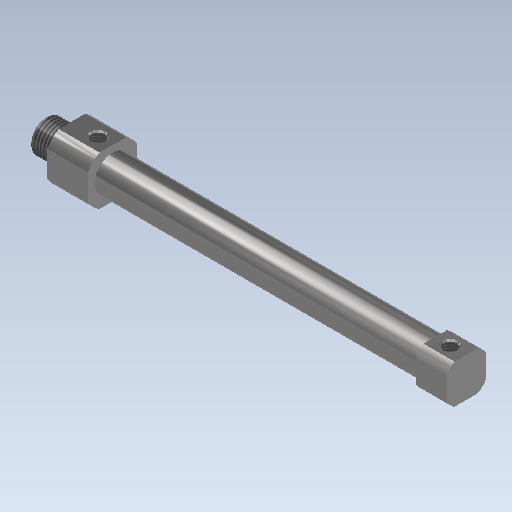
# Autodesk Inventor part: CJ2KB10-75Z(0)_BODY
Saved by Autodesk Inventor 2021.3 (Build 253353010, 353A)
## iProperties
Created: 2019-10-24
Part Number: CJ2KB10-75Z(0)_BODY
Material: ステンレス鋼
Catalog Web Link: www.cadenas.de
Description: CJ2K-Z_BODY-Air Cylinder/Non-rotating Rod Type: Double Acting, Single Rod
Vendor: SMC
Document SubType Name: Modeling
Designer: psadmin
Manufacturer: SMC
Mass: 57.0241 g
Surface Area: 82.6037 cm^2
Volume: 7.12801 cm^3
Density: 8 g/cm^3
Appearance: 半つや出し
Category: PARTsolutions
Company: SMC
PSOL_IDENT_0: {$CADENAS_DATA\23d-libs\smc_jp\actuator\standard_air_cylinder\cj2\cj2k_z\parts\cj2k_z_body.prj},256
PSOL_IDENT_1: {VTYP=3D},{NB=CJ2KB10-75Z(0)_BODY},{LINA=CJ2KB10-75Z_BODY},{NN=CJ2K-Z_BODY},{DATE=07.02.2019 07:32:0
PSOL_IDENT_2: 0},{GEOMDATE=05.03.2018 07:17:00},{VERSION=},{LINEID=370},{WBVAR=MAGNET,AUTOSWITCH,NUMBER,STROKE,POR
PSOL_IDENT_3: T,MOUNTING,OMSCXC3,OMSCXC51,THREAD},{WBNUMERIC=STROKE}  {NB=CJ2KB10-75Z(0)_BODY},{LINA=CJ2KB10-75Z_B
PSOL_IDENT_4: ODY},{KT=DUMMY},{ORDER=CJ2KB10-75Z},{BORE=10},{MOUNT=(B) Basic},{MAGNET=},{MOUNTX=B},{AUTOSWITCH=},{
PSOL_IDENT_5: NUMBER=},{STROKE=75},{SMAX=400},{PORT=},{PORTX='', '(-) Perpendicular', 'R', '(R) In-line'},{MOUNTIN
PSOL_IDENT_6: G=},{MOUNTINGX='','N/A'},{OMSCXC3=},{OMSCXC51=},{THREAD=0},{BA=15.0},{BB=12.0},{CA=17.0},{CB=14.0},{
PSOL_IDENT_7: CD=0.0},{CX=0.0},{F=8},{GA=8.0},{GB=5.0},{H=28},{KA=4.2},{NA=12.5},{NB1=9.5},{NDH8=10 0/-0.022},{NN=
PSOL_IDENT_8: M10x1.0},{NN1=10},{NN2=1.0},{R=0},{S=46},{U=0},{RAIL=off},{AUTOSWX='','N/A'},{SW=4.5},{SWX=4.5},{SW1=
PSOL_IDENT_9: 6.000},{SW2=2.000},{SW3=2.500},{SW4=1.500},{SW5=4.500},{SW6=0.500},{SW7=3.000},{SW8=3.500},{SW9=0.50
PSOL_IDENT_10: 0},{SWSIGNX= '','N/A' },{XC3= '','(-) None','-XC3AB','(XC3AB) Special Port Location (Rod port locati
PSOL_IDENT_11: on: A,Head port location: B)','-XC3AC','(XC3AC) Special Port Location (Rod port location: A,Head por
PSOL_IDENT_12: t location: C)','-XC3AD','(XC3AD) Special Port Location (Rod port location: A,Head port location: D)'
PSOL_IDENT_13: ,'-XC3BA','(XC3BA) Special Port Location (Rod port location: B,Head port location: A)','-XC3BB','(XC
PSOL_IDENT_14: 3BB) Special Port Location (Rod port location: B,Head port location: B)','-XC3BC','(XC3BC) Special P
PSOL_IDENT_15: ort Location (Rod port location: B,Head port location: C)','-XC3BD','(XC3BD) Special Port Location (
PSOL_IDENT_16: Rod port location: B,Head port location: D)','-XC3CA','(XC3CA) Special Port Location (Rod port locat
PSOL_IDENT_17: ion: C,Head port location: A)','-XC3CB','(XC3CB) Special Port Location (Rod port location: C,Head po
PSOL_IDENT_18: rt location: B)','-XC3CC','(XC3CC) Special Port Location (Rod port location: C,Head port location: C
PSOL_IDENT_19: )','-XC3CD','(XC3CD) Special Port Location (Rod port location: C,Head port location: D)','-XC3DA','(
PSOL_IDENT_20: XC3DA) Special Port Location (Rod port location: D,Head port location: A)','-XC3DB','(XC3DB) Special
PSOL_IDENT_21: Port Location (Rod port location: D,Head port location: B)','-XC3DC','(XC3DC) Special Port Location
PSOL_IDENT_22: (Rod port location: D,Head port location: C)','-XC3DD','(XC3DD) Special Port Location (Rod port loc
PSOL_IDENT_23: ation: D,Head port location: D)' },{XC51= '','(-) None','-XC51H4','(XC51H4) Hose nipple type: ø4/2.5
PSOL_IDENT_24: with restriction','-XC51H6','(XC51H6) Hose nipple type: ø6/4 with restriction','-XC51MH4','(XC51MH4
PSOL_IDENT_25: ) Hose nipple type: ø4/2.5 without restriction','-XC51MH6','(XC51MH6) Hose nipple type: ø6/4 without
PSOL_IDENT_26: restriction' },{PORTXC3=A1},{PORTXC32=A2},{MODEL=M-5H-6}
NN: M10x1.0
NT: Air Cylinder/Non-rotating Rod Type: Double Acting, Single Rod
NB: CJ2KB10-75Z(0)_BODY
NBSYN: $ORDER.($THREAD.)_BODY
LINA: CJ2KB10-75Z_BODY
BORE: 10
MOUNT: (B) Basic
MAGNET: (-) Without magnet
AUTOSWITCH: N/A
NUMBER: N/A
STROKE: 75
SMAX: 400
PORT: (-) Perpendicular
MOUNTING: N/A
OMSCXC3: (-) None
OMSCXC51: (-) None
THREAD: on
BA: 15
BB: 12
CA: 17
CB: 14
CD: 0
CX: 0
F: 8
GA: 8
GB: 5
H: 28
KA: 4.2
NA: 12.5
NB1: 9.5
NDH8: 10 0/-0.022
NN1: 10
NN2: 1
R: 0
S: 46
U: 0
RAIL: off
SW1: 6
SW2: 2
SW3: 2.5
SW4: 1.5
SW5: 4.5
SW6: 0.5
SW7: 3
SW8: 3.5
SW9: 0.5
SUPPLIER: SMC
ARTICLENO: CJ2KB10-75Z(0)_BODY
BOMINFO: CJ2KB10-75Z_BODY
CREATOR: CADENAS GmbH
Title: CJ2KB10-75Z_BODY
Author: Cadenas PARTsolutions
Comments: Air Cylinder/Non-rotating Rod Type: Double Acting, Single Rod
Autodesk Inventor part; units mm, degrees
sketch "Sketch_8" plane through (0, 0, 0) normal (0, 0, 1) x (1, 0, 0)
  line L0 (0, 0) -> (-8, 0)
  line L1 (-8, 0) -> (-8, 4.4585)
  line L2 (-8, 4.4585) -> (-7.4585, 5)
  line L3 (-7.4585, 5) -> (0, 5)
  line L4 (0, 5) -> (0, 0)
  line L5 (0, 0) -> (-8, 0)
  constraints: 12 end point
revolve "Revolution1" add sketch "Sketch_8" angle 360 about axis through (0, 0, 0) along (1, 0, 0)
thread "Thread1" size "M10x1" class "6g" standard "ISO Metric profile" length 5.9585
sketch "Sketch_9" plane through (0, 0, 0) normal (1, 0, 0) x (0, 0, -1)
  line L0 (-7.5, 4) -> (-7.5, -4)
  arc A0 (-7.5, -4) -> (-4, -7.5) centre (0, 0) ccw
  line L1 (-4, -7.5) -> (4, -7.5)
  arc A1 (4, -7.5) -> (7.5, -4) centre (0, 0) ccw
  line L2 (7.5, -4) -> (7.5, 4)
  arc A2 (7.5, 4) -> (4, 7.5) centre (0, 0) ccw
  line L3 (4, 7.5) -> (-4, 7.5)
  arc A3 (-4, 7.5) -> (-7.5, 4) centre (0, 0) ccw
  constraints: 8 end point, 8 point on circle, 4 centre point
extrude "Extrusion1" add sketch "Sketch_9" along normal blind 12.5
sketch "Sketch_6" plane through (12.5, 0, 0) normal (1, 0, 0) x (0, 0, -1)
  circle A0 centre (0, 0) radius 5.5
  constraints: 1 centre point
extrude "Extrusion2" add sketch "Sketch_6" along normal blind 99
sketch "Sketch_10" plane through (111.5, 0, 0) normal (1, 0, 0) x (0, 0, -1)
  line L0 (-6, 3.6056) -> (-6, -3.6056)
  arc A0 (-6, -3.6056) -> (-3.6056, -6) centre (0, 0) ccw
  line L1 (-3.6056, -6) -> (3.6056, -6)
  arc A1 (3.6056, -6) -> (6, -3.6056) centre (0, 0) ccw
  line L2 (6, -3.6056) -> (6, 3.6056)
  arc A2 (6, 3.6056) -> (3.6056, 6) centre (0, 0) ccw
  line L3 (3.6056, 6) -> (-3.6056, 6)
  arc A3 (-3.6056, 6) -> (-6, 3.6056) centre (0, 0) ccw
  constraints: 8 end point, 8 point on circle, 4 centre point
extrude "Extrusion3" add sketch "Sketch_10" along normal blind 9.5
sketch "Sketch5" plane through (0, 7.5, 4) normal (0, 1, 0) x (1, 0, 0)
  point P0 (8, 4)
hole "Hole1" at (8, 7.5, 0) direction (0, -1, 0) diameter 4.134 depth 5.5 tip angle 150 countersink diameter 5 countersink angle 90 thread size "M5x0.8" class "6H" standard "ISO Metric profile"
sketch "Sketch6" plane through (111.5, 6, 3.6056) normal (0, 1, 0) x (1, 0, 0)
  point P0 (4.5, 3.6056)
hole "Hole2" at (116, 6, 0) direction (0, -1, 0) diameter 4.134 depth 5.5 tip angle 150 countersink diameter 5 countersink angle 90 thread size "M5x0.8" class "6H" standard "ISO Metric profile"
sketch "Sketch_26" plane through (-8, 0, 0) normal (1, 0, 0) x (0, 0, -1)
  line L0 (-2.4249, 0) -> (-1.2124, -2.1)
  line L1 (-1.2124, -2.1) -> (1.2124, -2.1)
  line L2 (1.2124, -2.1) -> (2.4249, 0)
  line L3 (2.4249, 0) -> (1.2124, 2.1)
  line L4 (1.2124, 2.1) -> (-1.2124, 2.1)
  line L5 (-1.2124, 2.1) -> (-2.4249, 0)
  constraints: 12 end point
extrude "Extrusion4" cut sketch "Sketch_26" along normal blind 20.5
sketch "Sketch_16" plane through (0, 0, 0) normal (0, 0, 1) x (1, 0, 0)
  line L0 (92.5, 0) -> (12.5, 0)
  line L1 (12.5, 0) -> (12.5, 5)
  line L2 (12.5, 5) -> (92.5, 5)
  line L3 (92.5, 5) -> (92.5, 0)
  line L4 (92.5, 0) -> (12.5, 0)
  constraints: 10 end point
revolve "Revolution2" cut sketch "Sketch_16" angle 360 about axis through (92.5, 0, 0) along (1, 0, 0)
ref_plane "BODY_N_XY" through (121, 0, 0) normal (0, 0, 1) x (1, 0, 0)
ref_plane "BODY_N_YZ" through (121, 0, 0) normal (1, 0, 0) x (0, 1, 0)
ref_plane "BODY_N_ZX" through (121, 0, 0) normal (0, 1, 0) x (0, 0, 1)
ref_plane "BSW1_XY" through (17, 0, 0) normal (1, 0, 0) x (0, 0, -1)
ref_plane "BSW1_YZ" through (17, 0, 0) normal (0, 0, -1) x (0, 1, 0)
ref_plane "BSW1_ZX" through (17, 0, 0) normal (0, 1, 0) x (1, 0, 0)
ref_plane "BSW2_XY" through (107, 0, 0) normal (-1, 0, 0) x (0, 0, -1)
ref_plane "BSW2_YZ" through (107, 0, 0) normal (0, 0, -1) x (0, -1, 0)
ref_plane "BSW2_ZX" through (107, 0, 0) normal (0, -1, 0) x (-1, 0, 0)
ref_plane "RSW1_XY" through (17, -11, 0) normal (1, 0, 0) x (0, 0, -1)
ref_plane "RSW1_YZ" through (17, -11, 0) normal (0, 0, -1) x (0, 1, 0)
ref_plane "RSW1_ZX" through (17, -11, 0) normal (0, 1, 0) x (1, 0, 0)
ref_plane "RSW2_XY" through (107, -11, 0) normal (-1, 0, 0) x (0, 0, -1)
ref_plane "RSW2_YZ" through (107, -11, 0) normal (0, 0, -1) x (0, -1, 0)
ref_plane "RSW2_ZX" through (107, -11, 0) normal (0, -1, 0) x (-1, 0, 0)
ref_plane "body_XY" through (0, 0, 0) normal (1, 0, 0) x (0, 0, -1)
ref_plane "body_YZ" through (0, 0, 0) normal (0, 0, -1) x (0, 1, 0)
ref_plane "body_ZX" through (0, 0, 0) normal (0, 1, 0) x (1, 0, 0)
ref_plane "body2_XY" through (121, 0, 0) normal (-1, 0, 0) x (0, 0, -1)
ref_plane "body2_YZ" through (121, 0, 0) normal (0, 0, -1) x (0, -1, 0)
ref_plane "body2_ZX" through (121, 0, 0) normal (0, -1, 0) x (-1, 0, 0)
ref_plane "rod_XY" through (-28, 0, 0) normal (-1, 0, 0) x (0, 0, -1)
ref_plane "rod_YZ" through (-28, 0, 0) normal (0, 0, -1) x (0, -1, 0)
ref_plane "rod_ZX" through (-28, 0, 0) normal (0, -1, 0) x (-1, 0, 0)
body "Solid1"
